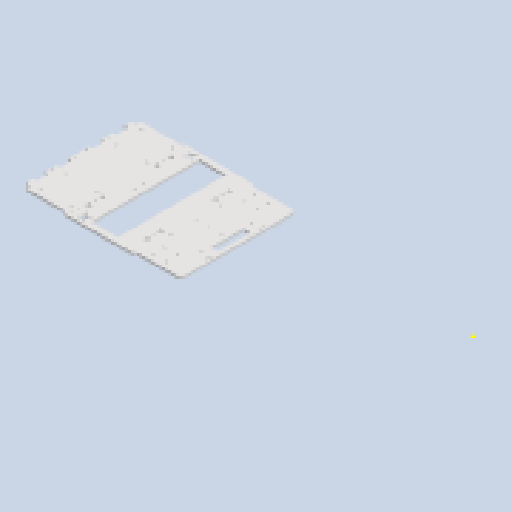
# Autodesk Inventor part: нижняя пластина
Saved by Autodesk Inventor 2024.2 (Build 282272000, 272)
## iProperties
Created: 2025-11-23
Part Number: нижняя пластина
Material: Типовые
Document SubType Name: Modeling
Designer: katya_notebook
Density: 1 g/cm^3
Appearance: По умолчанию
Author: katya_notebook
Autodesk Inventor part; units mm, degrees
(part 1 of 2)
ref_plane "YZ Plane" through (0, 0, 0) normal (1, 0, 0) x (0, 1, 0)
ref_plane "XZ Plane" through (0, 0, 0) normal (0, 1, 0) x (-1, 0, 0)
ref_plane "XY Plane" through (0, 0, 0) normal (0, 0, 1) x (1, 0, 0)
ref_plane "РабПлоскость1" through (-553.278877, -264.300199, 1.422232) normal (0, 1, 0) x (-1, 0, 0)
sketch "Эскиз1" plane through (-553.278877, -264.300199, 1.422232) normal (0, 1, 0) x (-1, 0, 0)
  line L0 (-30, 163.500004) -> (30, 163.500003)
  line L1 (-30, -31.5) -> (30, -31.5)
  line L2 (46.476267, 163.500003) -> (-223.523733, 163.500003)
  line L3 (-223.523733, 163.500003) -> (-223.523733, -31.5)
  line L4 (-223.523733, -31.5) -> (46.476267, -31.5)
  line L5 (46.476267, -31.5) -> (46.476267, 163.500003)
  point P0 (-553.278877, -1.422232)
  point P1 (-30, -30)
  point P2 (30, -30)
  point P3 (30, 162.000003)
  point P4 (-30, 162.000004)
  dimension "d1" = 270
  dimension "d6" = 0
  dimension "d7" = 0
  constraints: 8 end point, 2 coincident, 2 parallel, 1 horizontal, 1 perpendicular
  measures "d1" distance of L2.start L2.end
  measures "d6" distance from line of L4 L1.end
  measures "d7" distance from line of L2 L0.end
extrude "Выдавливание1" add sketch "Эскиз1" along normal blind 4
sketch "Эскиз2" plane through (-553.278877, -264.300199, 1.422232) normal (0, -1, 0) x (1, 0, 0)
  circle A0 centre (26, 108.500004) radius 2
  circle A1 centre (-26, 151.000003) radius 2
  circle A2 centre (26, 151.000004) radius 2
  circle A3 centre (-26, 108.500003) radius 2
  line L0 (-21.5, 122.000003) -> (-21.5, 157.000003)
  line L1 (-23.5, 122.000003) -> (-21.5, 122.000003)
  line L2 (-23.5, 157.000003) -> (-23.5, 122.000003)
  line L3 (-30, 157.000003) -> (-23.5, 157.000003)
  line L4 (-30, 157.000003) -> (-30, 103.500003)
  line L5 (-30, 103.500003) -> (30, 103.500004)
  line L6 (30, 103.500004) -> (30, 157.000004)
  line L7 (23.5, 157.000004) -> (30, 157.000004)
  line L8 (23.5, 122.000004) -> (23.5, 157.000004)
  line L9 (21.5, 122.000004) -> (23.5, 122.000004)
  line L10 (21.5, 157.000004) -> (21.5, 122.000004)
  line L11 (-21.5, 157.000003) -> (21.5, 157.000004)
  circle A4 centre (26, 23.5) radius 2
  circle A5 centre (-26, -19) radius 2
  circle A6 centre (26, -19) radius 2
  circle A7 centre (-26, 23.5) radius 2
  line L12 (-21.5, 10) -> (-21.5, -25)
  line L13 (-21.5, -25) -> (21.5, -25)
  line L14 (21.5, -25) -> (21.5, 10)
  line L15 (21.5, 10) -> (23.5, 10)
  line L16 (23.5, 10) -> (23.5, -25)
  line L17 (23.5, -25) -> (30, -25)
  line L18 (30, 28.5) -> (30, -25)
  line L19 (-30, 28.5) -> (30, 28.5)
  line L20 (-30, -25) -> (-30, 28.5)
  line L21 (-30, -25) -> (-23.5, -25)
  line L22 (-23.5, -25) -> (-23.5, 10)
  line L23 (-23.5, 10) -> (-21.5, 10)
  circle A8 centre (26, -19) radius 2
  circle A9 centre (26, 23.5) radius 2
  circle A10 centre (-26, -19) radius 2
  circle A11 centre (-26, 23.5) radius 2
  circle A12 centre (26, 108.500004) radius 2
  circle A13 centre (26, 151.000004) radius 2
  circle A14 centre (-26, 108.500003) radius 2
  circle A15 centre (-26, 151.000003) radius 2
  point P0 (553.278877, -1.422232)
  constraints: 8 centre point, 8 coincident, 8 concentric
extrude "Выдавливание2" cut sketch "Эскиз2" against normal blind 4 contours A0 | A1 | A2 | A3 | A4 | A5 | A6 | A7
sketch "Эскиз3" plane through (-553.278877, -264.300199, 1.422232) normal (0, -1, 0) x (1, 0, 0)
  spline S0 degree 3 poles (167.530647, -1.5) (167.530647, -1.675228) (167.505938, -1.863112) (167.406969, -2.216269) (167.332996, -2.381628) (167.143154, -2.701977) (167.002629, -2.869355) (166.694843, -3.139058) (166.528045, -3.241917) (165.99333, -3.490366) (165.589204, -3.533982) (164.848659, -3.417135) (164.512124, -3.257434) (164.024214, -2.845742) (163.799855, -2.568258) (163.628417, -2.126382) (163.592902, -2.011125) (163.543842, -1.762124) (163.530647, -1.627897) (163.530647, -1.372102) (163.543842, -1.237875) (163.592902, -0.988874) (163.628417, -0.873617) (163.799855, -0.431742) (164.024214, -0.154257) (164.512124, 0.257435) (164.848659, 0.417136) (165.589204, 0.533983) (165.99333, 0.490367) (166.528045, 0.241918) (166.694843, 0.139059) (167.002629, -0.130644) (167.143154, -0.298022) (167.332996, -0.618371) (167.406969, -0.78373) (167.505938, -1.136887) (167.530647, -1.324772) (167.530647, -1.5) knots -1.5971811 -1.5971811 -1.5971811 -1.5971811 -1.5446127 -1.5446127 -1.49204429 -1.49204429 -1.42257961 -1.42257961 -1.35311492 -1.35311492 -1.18239978 -1.18239978 -1.01168465 -1.01168465 -0.87532923 -0.87532923 -0.83695989 -0.83695989 -0.79859055 -0.79859055 -0.76022121 -0.76022121 -0.72185188 -0.72185188 -0.58549645 -0.58549645 -0.41478132 -0.41478132 -0.24406618 -0.24406618 -0.17460149 -0.17460149 -0.10513681 -0.10513681 -0.0525684 -0.0525684 0 0 0 0
  spline S1 degree 3 poles (190.047468, -1.5) (190.047468, -1.620288) (190.036518, -1.738724) (189.995823, -1.966144) (189.966063, -2.075131) (189.855778, -2.381563) (189.753425, -2.558671) (189.3863, -3.048352) (189.043184, -3.281704) (188.267032, -3.529213) (187.832995, -3.536652) (187.236348, -3.337829) (187.042108, -3.243447) (186.680736, -2.977295) (186.514082, -2.804962) (186.286366, -2.464282) (186.197167, -2.285548) (186.077558, -1.900195) (186.047468, -1.693486) (186.047468, -1.306513) (186.077558, -1.099804) (186.197167, -0.714451) (186.286366, -0.535718) (186.514082, -0.195037) (186.680736, -0.022705) (187.042108, 0.243448) (187.236348, 0.33783) (187.832995, 0.536653) (188.267032, 0.529214) (189.043184, 0.281704) (189.3863, 0.048353) (189.753425, -0.441328) (189.855778, -0.618437) (189.966063, -0.924868) (189.995823, -1.033855) (190.036518, -1.261275) (190.047468, -1.379712) (190.047468, -1.5) knots -1.53992103 -1.53992103 -1.53992103 -1.53992103 -1.50383465 -1.50383465 -1.46774826 -1.46774826 -1.39557548 -1.39557548 -1.21717391 -1.21717391 -1.03877234 -1.03877234 -0.96241242 -0.96241242 -0.88605249 -0.88605249 -0.8280065 -0.8280065 -0.76996052 -0.76996052 -0.71191453 -0.71191453 -0.65386854 -0.65386854 -0.57750862 -0.57750862 -0.50114869 -0.50114869 -0.32274712 -0.32274712 -0.14434556 -0.14434556 -0.07217278 -0.07217278 -0.03608639 -0.03608639 0 0 0 0
  circle A0 centre (203.047466, 23.5) radius 2
  circle A1 centre (151.047466, 23.5) radius 2
  line L0 (206.802962, 28.5) -> (146.802962, 28.5)
  line L1 (146.802962, 28.5) -> (146.802962, -25)
  line L2 (206.802962, -25) -> (206.802962, 28.5)
  line L3 (197.047468, -6.5) -> (197.047468, -25)
  line L4 (157.047468, -25) -> (157.047468, -6.5)
  line L5 (157.047468, -6.5) -> (197.047468, -6.5)
  circle A2 centre (203.047467, -19) radius 2
  circle A3 centre (151.047467, -19) radius 2
  line L6 (197.047468, -25) -> (206.802962, -25)
  line L7 (146.802962, -25) -> (157.047468, -25)
  point P0 (553.278877, -1.422232)
  point P1 (167.530647, -1.5)
  point P2 (190.047468, -1.5)
  point P3 (201.315416, -20)
  point P4 (204.779518, -20)
  point P5 (149.315416, -20)
  point P6 (152.779518, -20)
extrude "Выдавливание3" cut sketch "Эскиз3" against normal blind 10 contours S0 | S1 | A0 | A1
sketch "Эскиз4" plane through (-553.278877, -264.300199, 1.422232) normal (0, -1, 0) x (1, 0, 0)
  circle A0 centre (151.047466, 108.500004) radius 2
  circle A1 centre (203.047466, 108.500003) radius 2
  spline S0 degree 3 poles (190.047468, 133.500003) (190.047468, 133.620291) (190.036518, 133.738728) (189.995823, 133.966148) (189.966063, 134.075135) (189.855778, 134.381566) (189.753425, 134.558675) (189.3863, 135.048356) (189.043184, 135.281707) (188.267032, 135.529217) (187.832995, 135.536656) (187.236348, 135.337833) (187.042108, 135.243451) (186.680736, 134.977298) (186.514082, 134.804966) (186.286366, 134.464285) (186.197167, 134.285552) (186.077558, 133.900199) (186.047468, 133.69349) (186.047468, 133.306517) (186.077558, 133.099808) (186.197167, 132.714455) (186.286366, 132.535721) (186.514082, 132.195041) (186.680736, 132.022708) (187.042108, 131.756556) (187.236348, 131.662174) (187.832995, 131.46335) (188.267032, 131.47079) (189.043184, 131.718299) (189.3863, 131.95165) (189.753425, 132.441332) (189.855778, 132.61844) (189.966063, 132.924872) (189.995823, 133.033859) (190.036518, 133.261279) (190.047468, 133.379715) (190.047468, 133.500003) knots 0 0 0 0 0.03608639 0.03608639 0.07217278 0.07217278 0.14434556 0.14434556 0.32274712 0.32274712 0.50114869 0.50114869 0.57750862 0.57750862 0.65386854 0.65386854 0.71191453 0.71191453 0.76996052 0.76996052 0.8280065 0.8280065 0.88605249 0.88605249 0.96241242 0.96241242 1.03877234 1.03877234 1.21717391 1.21717391 1.39557548 1.39557548 1.46774826 1.46774826 1.50383465 1.50383465 1.53992103 1.53992103 1.53992103 1.53992103
  spline S1 degree 3 poles (167.530647, 133.500003) (167.530647, 133.675231) (167.505938, 133.863116) (167.406969, 134.216273) (167.332996, 134.381632) (167.143154, 134.701981) (167.002629, 134.869359) (166.694843, 135.139062) (166.528045, 135.241921) (165.99333, 135.49037) (165.589204, 135.533986) (164.848659, 135.417139) (164.512124, 135.257438) (164.024214, 134.845746) (163.799855, 134.568261) (163.628417, 134.126386) (163.592902, 134.011129) (163.543842, 133.762128) (163.530647, 133.627901) (163.530647, 133.372105) (163.543842, 133.237879) (163.592902, 132.988878) (163.628417, 132.873621) (163.799855, 132.431745) (164.024214, 132.154261) (164.512124, 131.742569) (164.848659, 131.582868) (165.589204, 131.466021) (165.99333, 131.509637) (166.528045, 131.758086) (166.694843, 131.860945) (167.002629, 132.130648) (167.143154, 132.298026) (167.332996, 132.618375) (167.406969, 132.783734) (167.505938, 133.136891) (167.530647, 133.324775) (167.530647, 133.500003) knots 0 0 0 0 0.0525684 0.0525684 0.10513681 0.10513681 0.17460149 0.17460149 0.24406618 0.24406618 0.41478132 0.41478132 0.58549645 0.58549645 0.72185188 0.72185188 0.76022121 0.76022121 0.79859055 0.79859055 0.83695989 0.83695989 0.87532923 0.87532923 1.01168465 1.01168465 1.18239978 1.18239978 1.35311492 1.35311492 1.42257961 1.42257961 1.49204429 1.49204429 1.5446127 1.5446127 1.5971811 1.5971811 1.5971811 1.5971811
  circle A2 centre (151.047467, 151.000004) radius 2
  circle A3 centre (203.047467, 151.000003) radius 2
  point P0 (553.278877, -1.422232)
  point P1 (190.047468, 133.500003)
  point P2 (167.530647, 133.500003)
  point P3 (149.315416, 152.000003)
  point P4 (152.779518, 152.000003)
  point P5 (201.315416, 152.000003)
  point P6 (204.779518, 152.000003)
extrude "Выдавливание4" cut sketch "Эскиз4" against normal blind 10 contours A0 | A1 | S0 | S1
sketch "Эскиз6" plane through (-553.278877, -264.300199, 1.422232) normal (0, -1, 0) x (1, 0, 0)
  circle A0 centre (53.523733, 156.000002) radius 5
  circle A1 centre (53.523733, 156.000002) radius 2.5
  circle A2 centre (53.523733, 156.000002) radius 5
  circle A3 centre (53.523733, -23.999998) radius 5
  circle A4 centre (53.523733, -23.999998) radius 5
  point P0 (553.278877, -1.422232)
  constraints: 2 centre point, 2 coincident, 2 concentric
extrude "Выдавливание6" cut sketch "Эскиз6" against normal blind 10 contours A0 | A1 | A3
sketch "Эскиз7" plane through (-553.278877, -264.300199, 1.422232) normal (0, -1, 0) x (1, 0, 0)
  line L0 (30, 103.500004) -> (30, 157.000004)
  line L1 (-46.476267, 163.500003) -> (223.523733, 163.500003)
  line L2 (30.270127, 167.770131) -> (146.697322, 167.770131)
  line L3 (146.802962, 163.500003) -> (146.802962, 157.000003)
  line L4 (146.802962, 167.770131) -> (146.697322, 167.770131)
  line L5 (146.802962, 163.500003) -> (30, 163.500003)
  line L6 (30.000003, 28.5) -> (30.000003, -25)
  line L7 (30.000003, -25) -> (30.000003, -31.5)
  line L8 (146.802962, -31.5) -> (146.802962, -25)
  line L9 (146.802962, -35.5) -> (30.000003, -35.5)
  line L10 (30.000003, -31.5) -> (146.802962, -31.5)
  line L11 (30, 163.500003) -> (26, 163.500003)
  arc A0 (26, 163.500003) -> (30.270127, 167.770131) centre (22.8966, 170.873531) ccw
  line L12 (146.802962, 163.500003) -> (150.802962, 163.500003)
  arc A1 (146.802962, 167.770131) -> (150.802962, 163.500003) centre (154.237087, 170.72543) ccw
  line L13 (30.000003, -31.5) -> (26.000003, -31.5)
  line L14 (223.523733, -31.5) -> (-46.476267, -31.5)
  arc A2 (30.000003, -35.5) -> (26.000003, -31.5) centre (22.7085, -38.791502) ccw
  line L15 (146.802962, -31.5) -> (150.802962, -31.5)
  arc A3 (150.802962, -31.5) -> (146.802962, -35.5) centre (154.094465, -38.791502) ccw
  point P0 (553.278877, -1.422232)
  dimension "d23" = 8
  dimension "d24" = 8
  dimension "d26" = 8
  dimension "d28" = 8
  constraints: 18 end point, 8 point on circle, 5 point on line, 4 centre point, 2 collinear, 1 parallel
  measures "d23" radius of A0
  measures "d24" radius of A1
  measures "d26" radius of A2
  measures "d28" radius of A3
extrude "Выдавливание7" add sketch "Эскиз7" against normal blind 4
sketch "Эскиз8" plane through (-553.278877, -264.300199, 1.422232) normal (0, -1, 0) x (1, 0, 0)
  circle A0 centre (57.777238, 162.775524) radius 1.5
  circle A1 centre (60.299256, 151.746498) radius 1.5
  circle A2 centre (49.270229, 149.22448) radius 1.5
  circle A3 centre (46.748211, 160.253506) radius 1.5
  circle A4 centre (57.777238, 162.775524) radius 1.5
  circle A5 centre (60.299256, 151.746498) radius 1.5
  circle A6 centre (49.270229, 149.22448) radius 1.5
  circle A7 centre (46.748211, 160.253506) radius 1.5
  circle A8 centre (60.299256, -19.746494) radius 1.5
  circle A9 centre (57.777238, -30.775521) radius 1.5
  circle A10 centre (46.748211, -28.253503) radius 1.5
  circle A11 centre (49.270229, -17.224476) radius 1.5
  circle A12 centre (49.270229, -17.224476) radius 1.5
  circle A13 centre (60.299256, -19.746494) radius 1.5
  circle A14 centre (57.777238, -30.775521) radius 1.5
  circle A15 centre (46.748211, -28.253503) radius 1.5
  point P0 (553.278877, -1.422232)
  constraints: 8 centre point, 8 coincident, 8 concentric
extrude "Выдавливание8" cut sketch "Эскиз8" against normal blind 4
sketch "Эскиз9" plane through (-553.278877, -264.300199, 1.422232) normal (0, -1, 0) x (1, 0, 0)
  line L0 (223.523733, 163.500003) -> (223.523733, -31.5)
  line L1 (-46.476267, -31.5) -> (-46.476267, 163.500003)
  line L2 (223.523733, 163.500003) -> (-46.476267, 163.500003)
  line L3 (-46.476267, 163.500003) -> (-46.476267, -31.5)
  line L4 (-46.476267, -31.5) -> (223.523733, -31.5)
  line L5 (223.523733, -31.5) -> (223.523733, 163.500003)
  line L6 (223.523733, 66.000002) -> (-46.476267, 66.000002)
  line L7 (88.523733, 163.500003) -> (88.523733, -31.5)
  line L8 (66.023733, -25.499998) -> (111.023733, -25.499998)
  line L9 (111.023733, -25.499998) -> (111.023733, 157.500002)
  line L10 (111.023733, 157.500002) -> (66.023733, 157.500002)
  line L11 (66.023733, 157.500002) -> (66.023733, -25.499998)
  line L12 (66.023733, -25.499998) -> (111.023733, 157.500002) construction
  line L13 (111.023733, -25.499998) -> (66.023733, 157.500002) construction
  point P0 (553.278877, -1.422232)
  point P1 (88.523733, 66.000002)
  dimension "d33" = 183
  dimension "d34" = 45
  constraints: 24 end point, 7 midpoint, 4 parallel, 2 horizontal, 2 perpendicular
  measures "d33" distance of L8.end L9.end
  measures "d34" distance of L9.end L10.end
extrude "Выдавливание9" cut sketch "Эскиз9" against normal blind 4 contours L9 L8 L7 L6 | L6 L7 L10 L9 | L7 L6 L11 L10 | L7 L8 L11 L6
sketch "Эскиз10" plane through (-553.278877, -264.300199, 1.422232) normal (0, -1, 0) x (1, 0, 0)
  line L0 (36.973733, 147.850002) -> (34.973733, 147.850002)
  line L1 (36.973733, 147.850002) -> (36.973733, 152.650002)
  line L2 (35.973733, 147.850002) -> (35.973733, 152.650002)
  line L3 (36.973733, 159.350002) -> (34.973733, 159.350002)
  line L4 (36.973733, 150.250002) -> (34.973733, 150.250002)
  line L5 (36.973733, 159.350002) -> (36.973733, 164.150002)
  line L6 (36.973733, 161.750002) -> (33.994288, 161.750002)
  line L7 (33.994288, 161.750002) -> (35.973733, 159.350002)
  line L8 (35.973733, 164.150002) -> (35.973733, 159.350002)
  circle A0 centre (35.973733, 161.750002) radius 1
  circle A1 centre (35.973733, 150.250002) radius 1
  point P0 (553.278877, -1.422232)
  point P1 (34.973733, 147.000002)
  point P2 (30, 163.500005)
  point P3 (34.973733, 161.750002)
  point P4 (35.973733, 162.750002)
  point P5 (35.973733, 161.750002)
  constraints: 18 end point, 4 midpoint, 4 perpendicular, 2 horizontal, 1 horizontal alignment, 6 other
extrude "Выдавливание10" cut sketch "Эскиз10" against normal blind 10 contours A1 L2 L4 | L4 L2 A1 | A1 L4 L2 | L4 A1 L2 | A0 L8 L6 | L6 L8 A0 | A0 L6 L8 | L6 A0 L8
sketch "Эскиз11" plane through (-553.278877, -264.300199, 1.422232) normal (0, -1, 0) x (1, 0, 0)
  arc A0 (34.973733, -29.749998) -> (36.973733, -29.749998) centre (35.973733, -29.749998) ccw
  arc A1 (36.973733, -29.749998) -> (34.973733, -29.749998) centre (35.973733, -29.749998) ccw
  arc A2 (34.973733, -18.249998) -> (36.973733, -18.249998) centre (35.973733, -18.249998) ccw
  arc A3 (36.973733, -18.249998) -> (34.973733, -18.249998) centre (35.973733, -18.249998) ccw
  point P0 (553.278877, -1.422232)
extrude "Выдавливание11" cut sketch "Эскиз11" against normal blind 10
sketch "Эскиз12" plane through (-553.278877, -264.300199, 1.422232) normal (0, -1, 0) x (1, 0, 0)
  circle A0 centre (55.548733, 57.85394) radius 2
  circle A1 centre (55.548733, 73.85394) radius 2
  point P0 (553.278877, -1.422232)
extrude "Выдавливание12" cut sketch "Эскиз12" against normal blind 10
sketch "Эскиз13" plane through (-553.278877, -264.300199, 1.422232) normal (0, -1, 0) x (1, 0, 0)
  point P0 (553.278877, -1.422232)
sketch "Эскиз14" plane through (-553.278877, -264.300199, 1.422232) normal (0, -1, 0) x (1, 0, 0)
  circle A0 centre (217.523733, 18.5) radius 2
  circle A1 centre (217.523733, 113.500003) radius 2
  line L0 (150.802962, 163.500003) -> (223.523733, 163.500003)
  line L1 (223.523733, -31.5) -> (150.802962, -31.5)
  line L2 (223.523733, 163.500003) -> (223.523733, -31.5)
  circle A2 centre (217.523733, 24.5) radius 2
  circle A3 centre (217.523733, 107.500003) radius 2
  point P0 (553.278877, -1.422232)
  dimension "d43" = 4
  dimension "d44" = 4
  dimension "d45" = 50
  dimension "d46" = 50
  dimension "d47" = 6
  dimension "d48" = 6
  dimension "d51" = 4
  dimension "d52" = 6
  dimension "d53" = 6
  dimension "d54" = 4
  dimension "d55" = 6
  dimension "d56" = 6
  constraints: 4 centre point
  measures "d43" diameter of A1
  measures "d44" diameter of A0
  measures "d45" distance from line of L0 A1.centre
  measures "d46" distance from line of L1 A0.centre
  measures "d47" distance from line of L2 A0.centre
  measures "d48" distance from line of L2 A1.centre
  measures "d51" diameter of A3
  measures "d52" distance of A1.centre A3.centre
  measures "d53" distance from line of L2 A3.centre
  measures "d54" diameter of A2
  measures "d55" distance from line of L2 A2.centre
  measures "d56" distance of A0.centre A2.centre
extrude "Выдавливание13" cut sketch "Эскиз14" against normal blind 10
sketch "Эскиз15" plane through (-553.278877, -264.300199, 1.422232) normal (0, -1, 0) x (1, 0, 0)
  line L0 (216.523733, 93.576493) -> (204.523733, 93.576493)
  line L1 (204.523733, 93.576493) -> (204.523733, 38.576493)
  line L2 (204.523733, 38.576493) -> (216.523733, 38.576493)
  line L3 (216.523733, 38.576493) -> (216.523733, 93.576493)
  line L4 (216.523733, 93.576493) -> (204.523733, 38.576493) construction
  line L5 (204.523733, 93.576493) -> (216.523733, 38.576493) construction
  line L6 (223.523733, 163.500003) -> (223.523733, -31.5)
  point P0 (553.278877, -1.422232)
  point P1 (210.523733, 66.076493)
  dimension "d57" = 13
  dimension "d58" = 12
  dimension "d59" = 55
  constraints: 12 end point, 2 midpoint, 2 parallel, 1 horizontal, 1 perpendicular
  measures "d57" distance from line of point (210.524, 66.076) L6
  measures "d58" distance of L0.start L0.end
  measures "d59" distance of L0.end L1.end
extrude "Выдавливание14" cut sketch "Эскиз15" against normal blind 10
sketch "Эскиз16" plane through (-553.278877, -264.300199, 1.422232) normal (0, -1, 0) x (1, 0, 0)
  spline S0 degree 3 poles (195.773733, 65.9) (195.773733, 66.088725) (195.735944, 66.289784) (195.582756, 66.659245) (195.467375, 66.827679) (195.201416, 67.093638) (195.03298, 67.209022) (194.663513, 67.362213) (194.462453, 67.4) (194.085014, 67.4) (193.883953, 67.362213) (193.514486, 67.209022) (193.346051, 67.093638) (193.080092, 66.827679) (192.964711, 66.659245) (192.811522, 66.289784) (192.773733, 66.088725) (192.773733, 65.711276) (192.811522, 65.510217) (192.964711, 65.140756) (193.080092, 64.972321) (193.346051, 64.706363) (193.514486, 64.590979) (193.883953, 64.437788) (194.085014, 64.4) (194.462453, 64.4) (194.663513, 64.437788) (195.03298, 64.590979) (195.201416, 64.706363) (195.467375, 64.972321) (195.582756, 65.140756) (195.735944, 65.510217) (195.773733, 65.711276) (195.773733, 65.9) knots -0.905867 -0.905867 -0.905867 -0.905867 -0.84924956 -0.84924956 -0.79263212 -0.79263212 -0.73601619 -0.73601619 -0.67940025 -0.67940025 -0.62278432 -0.62278432 -0.56616839 -0.56616839 -0.50955095 -0.50955095 -0.4529335 -0.4529335 -0.39631606 -0.39631606 -0.33969861 -0.33969861 -0.28308268 -0.28308268 -0.22646675 -0.22646675 -0.16985082 -0.16985082 -0.11323489 -0.11323489 -0.05661744 -0.05661744 0 0 0 0
  spline S1 degree 3 poles (172.273733, 66.1) (172.273733, 65.911276) (172.311522, 65.710217) (172.464711, 65.340756) (172.580092, 65.172321) (172.846051, 64.906363) (173.014486, 64.790979) (173.383953, 64.637788) (173.585014, 64.6) (173.962453, 64.6) (174.163513, 64.637788) (174.53298, 64.790979) (174.701416, 64.906363) (174.967375, 65.172321) (175.082756, 65.340756) (175.235944, 65.710217) (175.273733, 65.911276) (175.273733, 66.288725) (175.235944, 66.489784) (175.082756, 66.859245) (174.967375, 67.027679) (174.701416, 67.293638) (174.53298, 67.409022) (174.163513, 67.562213) (173.962453, 67.6) (173.585014, 67.6) (173.383953, 67.562213) (173.014486, 67.409022) (172.846051, 67.293638) (172.580092, 67.027679) (172.464711, 66.859245) (172.311522, 66.489784) (172.273733, 66.288725) (172.273733, 66.1) knots -0.905867 -0.905867 -0.905867 -0.905867 -0.84924956 -0.84924956 -0.79263212 -0.79263212 -0.73601619 -0.73601619 -0.67940025 -0.67940025 -0.62278432 -0.62278432 -0.56616839 -0.56616839 -0.50955095 -0.50955095 -0.4529335 -0.4529335 -0.39631606 -0.39631606 -0.33969861 -0.33969861 -0.28308268 -0.28308268 -0.22646675 -0.22646675 -0.16985082 -0.16985082 -0.11323489 -0.11323489 -0.05661744 -0.05661744 0 0 0 0
  spline S2 degree 3 poles (154.773733, 65.9) (154.773733, 66.088725) (154.735944, 66.289784) (154.582756, 66.659245) (154.467375, 66.827679) (154.201416, 67.093638) (154.03298, 67.209022) (153.663513, 67.362213) (153.462453, 67.4) (153.085014, 67.4) (152.883953, 67.362213) (152.514486, 67.209022) (152.346051, 67.093638) (152.080092, 66.827679) (151.964711, 66.659245) (151.811522, 66.289784) (151.773733, 66.088725) (151.773733, 65.711276) (151.811522, 65.510217) (151.964711, 65.140756) (152.080092, 64.972321) (152.346051, 64.706363) (152.514486, 64.590979) (152.883953, 64.437788) (153.085014, 64.4) (153.462453, 64.4) (153.663513, 64.437788) (154.03298, 64.590979) (154.201416, 64.706363) (154.467375, 64.972321) (154.582756, 65.140756) (154.735944, 65.510217) (154.773733, 65.711276) (154.773733, 65.9) knots -0.905867 -0.905867 -0.905867 -0.905867 -0.84924956 -0.84924956 -0.79263212 -0.79263212 -0.73601619 -0.73601619 -0.67940025 -0.67940025 -0.62278432 -0.62278432 -0.56616839 -0.56616839 -0.50955095 -0.50955095 -0.4529335 -0.4529335 -0.39631606 -0.39631606 -0.33969861 -0.33969861 -0.28308268 -0.28308268 -0.22646675 -0.22646675 -0.16985082 -0.16985082 -0.11323489 -0.11323489 -0.05661744 -0.05661744 0 0 0 0
  point P0 (553.278877, -1.422232)
  point P1 (195.773733, 65.9)
  point P2 (172.273733, 66.1)
  point P3 (154.773733, 65.9)
extrude "Выдавливание15" cut sketch "Эскиз16" against normal blind 10
sketch "Эскиз17" plane through (-553.278877, -260.300199, 1.422232) normal (0, 1, 0) x (1, 0, 0)
  line L0 (-46.476267, -143.500003) -> (-46.476267, -123.500003)
  line L1 (-46.476267, -143.500003) -> (-40.476267, -143.500003)
  line L2 (-40.476267, -123.500003) -> (-40.476267, -143.500003)
  line L3 (-46.476267, -123.500003) -> (-40.476267, -123.500003)
  line L4 (-46.476267, -103.500003) -> (-46.476267, -83.500003)
  line L5 (-46.476267, -103.500003) -> (-40.476267, -103.500003)
  line L6 (-40.476267, -83.500003) -> (-40.476267, -103.500003)
  line L7 (-46.476267, -83.500003) -> (-40.476267, -83.500003)
  line L8 (-46.476267, -48.5) -> (-46.476267, -28.5)
  line L9 (-46.476267, -48.5) -> (-40.476267, -48.5)
  line L10 (-40.476267, -28.5) -> (-40.476267, -48.5)
  line L11 (-46.476267, -28.5) -> (-40.476267, -28.5)
  line L12 (-46.476267, -8.5) -> (-46.476267, 11.5)
  line L13 (-46.476267, -8.5) -> (-40.476267, -8.5)
  line L14 (-40.476267, 11.5) -> (-40.476267, -8.5)
  line L15 (-46.476267, 11.5) -> (-40.476267, 11.5)
  circle A0 centre (-43.476267, -113.500003) radius 1.75
  circle A1 centre (-43.476267, -76.375003) radius 1.75
  circle A2 centre (-43.476267, -55.625003) radius 1.75
  circle A3 centre (-43.476267, -18.5) radius 1.75
  point P0 (553.278877, 1.422232)
extrude "Выдавливание16" cut sketch "Эскиз17" against normal blind 10
fillet "Сопряжение1" radius 8 4 edges at (-329.7551, -262.3002, -30.0778) (-329.7551, -262.3002, 164.9222) (-599.7551, -262.3002, -30.0778) (-599.7551, -262.3002, 164.9222)
sketch "Эскиз18" plane through (-599.755143, -264.300199, 104.922235) normal (-1, 0, 0) x (0, 0, 1)
  line L0 (-95.000003, 0) -> (-95.000003, 4)
  line L1 (-95.000003, 4) -> (-95.000003, 5)
  line L2 (-95.000003, 5) -> (-115.000003, 5)
  line L3 (-115.000003, 5) -> (-115.000003, 4)
  line L4 (-135.000003, 4) -> (-127.000003, 4)
  line L5 (-135.000003, 4) -> (-135.000003, -55.704973)
  line L6 (-115.000003, -55.704973) -> (-135.000003, -55.704973)
  line L7 (-115.000003, -55.704973) -> (-115.000003, -60.704973)
  line L8 (-115.000003, -60.704973) -> (-95.000003, -60.704973)
  line L9 (-95.000003, -60.704973) -> (-95.000003, -55.704973)
  line L10 (-86.750003, -55.704973) -> (-95.000003, -55.704973)
  line L11 (-86.750003, -55.704973) -> (-86.750003, -54.204972)
  line L12 (-86.750003, -54.204972) -> (-88.250003, -54.204972)
  line L13 (-88.250003, -54.204972) -> (-88.250003, -51.204972)
  line L14 (-88.250003, -51.204972) -> (-86.750003, -51.204972)
  line L15 (-86.750003, -51.204972) -> (-86.750003, -43.704972)
  line L16 (-86.750003, -43.704972) -> (-83.250003, -43.704972)
  line L17 (-83.250003, -43.704972) -> (-83.250003, -51.204972)
  line L18 (-83.250003, -51.204972) -> (-81.750003, -51.204972)
  line L19 (-81.750003, -51.204972) -> (-81.750003, -54.204972)
  line L20 (-81.750003, -54.204972) -> (-83.250003, -54.204972)
  line L21 (-83.250003, -54.204972) -> (-83.250003, -55.704973)
  line L22 (-75.000003, -55.704973) -> (-83.250003, -55.704973)
  line L23 (-75.000003, -55.704973) -> (-75.000003, -60.704973)
  line L24 (-75.000003, -60.704973) -> (-55.000003, -60.704972)
  line L25 (-55.000003, -60.704972) -> (-55.000003, -55.704972)
  line L26 (-49.624972, -55.704972) -> (-55.000003, -55.704972)
  line L27 (-49.624972, -55.704972) -> (-49.624972, -54.204972)
  line L28 (-49.624972, -54.204972) -> (-51.124972, -54.204972)
  line L29 (-51.124972, -54.204972) -> (-51.124972, -51.204972)
  line L30 (-51.124972, -51.204972) -> (-49.624972, -51.204972)
  line L31 (-49.624972, -51.204972) -> (-49.624972, -49.704972)
  line L32 (-49.624972, -49.704972) -> (-49.625, -49.704972)
  line L33 (-49.625, -49.704972) -> (-49.625, -43.704972)
  line L34 (-49.625, -43.704972) -> (-46.124972, -43.704972)
  line L35 (-46.124972, -43.704972) -> (-46.124972, -51.204972)
  line L36 (-46.124972, -51.204972) -> (-44.624972, -51.204972)
  line L37 (-44.624972, -51.204972) -> (-44.624972, -54.204972)
  line L38 (-44.624972, -54.204972) -> (-46.124972, -54.204972)
  line L39 (-46.124972, -54.204972) -> (-46.124972, -55.704972)
  line L40 (-28.875, -55.704972) -> (-46.124972, -55.704972)
  line L41 (-28.875, -55.704972) -> (-28.875, -54.204972)
  line L42 (-28.875, -54.204972) -> (-30.375, -54.204972)
  line L43 (-30.375, -54.204972) -> (-30.375, -51.204972)
  line L44 (-30.375, -51.204972) -> (-28.875, -51.204972)
  line L45 (-28.875, -51.204972) -> (-28.875, -43.704972)
  line L46 (-28.875, -43.704972) -> (-25.375, -43.704972)
  line L47 (-25.375, -43.704972) -> (-25.375, -51.204972)
  line L48 (-25.375, -51.204972) -> (-23.875, -51.204972)
  line L49 (-23.875, -51.204972) -> (-23.875, -54.204972)
  line L50 (-23.875, -54.204972) -> (-25.375, -54.204972)
  line L51 (-25.375, -54.204972) -> (-25.375, -55.704972)
  line L52 (-20, -55.704972) -> (-25.375, -55.704972)
  line L53 (-20, -55.704972) -> (-20, -60.704972)
  line L54 (-20, -60.704972) -> (0, -60.704972)
  line L55 (0, -60.704972) -> (0, -55.704972)
  line L56 (8.25, -55.704972) -> (0, -55.704972)
  line L57 (8.25, -55.704972) -> (8.25, -54.204972)
  line L58 (8.25, -54.204972) -> (6.75, -54.204972)
  line L59 (6.75, -54.204972) -> (6.75, -51.204972)
  line L60 (6.75, -51.204972) -> (8.25, -51.204972)
  line L61 (8.25, -51.204972) -> (8.25, -43.704972)
  line L62 (8.25, -43.704972) -> (11.75, -43.704972)
  line L63 (11.75, -43.704972) -> (11.75, -51.204972)
  line L64 (11.75, -51.204972) -> (13.25, -51.204972)
  line L65 (13.25, -51.204972) -> (13.25, -54.204972)
  line L66 (13.25, -54.204972) -> (11.75, -54.204972)
  line L67 (11.75, -54.204972) -> (11.75, -55.704972)
  line L68 (20, -55.704972) -> (11.75, -55.704972)
  line L69 (20, -55.704972) -> (20, -60.704972)
  line L70 (20, -60.704972) -> (40, -60.704972)
  line L71 (40, -60.704972) -> (40, -55.704972)
  line L72 (60, -55.704972) -> (40, -55.704972)
  line L73 (60, 4) -> (60, -55.704972)
  line L74 (52, 4) -> (60, 4)
  line L75 (40, 4) -> (40, 5)
  line L76 (40, 5) -> (20, 5)
  line L77 (20, 5) -> (20, 4)
  line L78 (20, 4) -> (20, 0)
  line L79 (20, 0) -> (13.25, 0)
  line L80 (13.25, 0) -> (13.25, -0.5)
  line L81 (13.25, -0.5) -> (11.75, -0.5)
  line L82 (11.75, -0.5) -> (11.75, -8)
  line L83 (11.75, -8) -> (8.25, -8)
  line L84 (8.25, -8) -> (8.25, -0.5)
  line L85 (8.25, -0.5) -> (6.75, -0.5)
  line L86 (6.75, -0.5) -> (6.75, 0)
  line L87 (6.75, 0) -> (0, 0)
  line L88 (0, 0) -> (0, 4)
  line L89 (0, 4) -> (0, 5)
  line L90 (0, 5) -> (-20, 5)
  line L91 (-20, 5) -> (-20, 4)
  line L92 (-20, 4) -> (-20, 0)
  line L93 (-20, 0) -> (-23.875, 0)
  line L94 (-23.875, 0) -> (-23.875, -0.5)
  line L95 (-23.875, -0.5) -> (-25.375, -0.5)
  line L96 (-25.375, -0.5) -> (-25.375, -8)
  line L97 (-25.375, -8) -> (-28.875, -8)
  line L98 (-28.875, -8) -> (-28.875, -0.5)
  line L99 (-28.875, -0.5) -> (-30.375, -0.5)
  line L100 (-30.375, -0.5) -> (-30.375, 0)
  line L101 (-30.375, 0) -> (-44.624972, 0)
  line L102 (-44.624972, 0) -> (-44.624972, -0.5)
  line L103 (-44.624972, -0.5) -> (-46.124972, -0.5)
  line L104 (-46.124972, -0.5) -> (-46.124972, -8)
  line L105 (-46.124972, -8) -> (-49.625, -8)
  line L106 (-49.625, -8) -> (-49.625, -2)
  line L107 (-49.625, -2) -> (-49.624972, -2)
  line L108 (-49.624972, -2) -> (-49.624972, -0.5)
  line L109 (-49.624972, -0.5) -> (-51.124972, -0.5)
  line L110 (-51.124972, -0.5) -> (-51.124972, 0)
  line L111 (-51.124972, 0) -> (-55.000003, 0)
  line L112 (-55.000003, 0) -> (-55.000003, 4)
  line L113 (-55.000003, 4) -> (-55.000003, 5)
  line L114 (-55.000003, 5) -> (-75.000003, 5)
  line L115 (-75.000003, 5) -> (-75.000003, 4)
  line L116 (-75.000003, 4) -> (-75.000003, 0)
  line L117 (-75.000003, 0) -> (-81.750003, 0)
  line L118 (-81.750003, 0) -> (-81.750003, -0.5)
  line L119 (-81.750003, -0.5) -> (-83.250003, -0.5)
  line L120 (-83.250003, -0.5) -> (-83.250003, -8)
  line L121 (-83.250003, -8) -> (-86.750003, -8)
  line L122 (-86.750003, -8) -> (-86.750003, -0.5)
  line L123 (-86.750003, -0.5) -> (-88.250003, -0.5)
  line L124 (-88.250003, -0.5) -> (-88.250003, 0)
  line L125 (-88.250003, 0) -> (-95.000003, 0)
  line L126 (52, 0) -> (-127.000003, 0)
  line L127 (52, 0) -> (52, 4)
  line L128 (52, 4) -> (60, 4)
  line L129 (60, 0) -> (60, 4)
  line L130 (60, 0) -> (52, 0)
  line L131 (-127.000003, 0) -> (-127.000003, 4)
  line L132 (-135.000003, 0) -> (-135.000003, 4)
  line L133 (-127.000003, 4) -> (-135.000003, 4)
  line L134 (-135.000003, 0) -> (-127.000003, 0)
  line L135 (-127.000003, 0) -> (-127.000003, 4)
  line L136 (52, 4) -> (52, 0)
  line L137 (52, 0) -> (40, 0)
  line L138 (40, 0) -> (40, 4)
  line L139 (-115.000003, 4) -> (-115.000003, 0)
  line L140 (-115.000003, 0) -> (-127.000003, 0)
  line L141 (-86.23393, -29.706046) -> (-86.23393, -22.248836)
  spline S0 degree 2 poles (-86.23393, -22.248836) (-86.23393, -21.656701) (-85.641794, -21.656701) knots 0 0 0 1 1 1
  spline S1 degree 2 poles (-85.641794, -21.656701) (-85.049659, -21.656701) (-85.049659, -22.248836) knots 0 0 0 1 1 1
  line L142 (-85.049659, -22.248836) -> (-85.049659, -29.11391)
  line L143 (-85.049659, -29.11391) -> (-83.624832, -29.11391)
  line L144 (-83.624832, -29.11391) -> (-82.051972, -22.054542)
  spline S2 degree 2 poles (-82.051972, -22.054542) (-81.95945, -21.656701) (-81.496844, -21.656701) knots 0 0 0 1 1 1
  spline S3 degree 2 poles (-81.496844, -21.656701) (-80.904709, -21.656701) (-80.904709, -22.230332) knots 0 0 0 1 1 1
  spline S4 degree 2 poles (-80.904709, -22.230332) (-80.904709, -22.304349) (-80.913961, -22.359862) knots 0 0 0 1 1 1
  line L145 (-80.913961, -22.359862) -> (-82.588595, -29.90034)
  spline S5 degree 2 poles (-82.588595, -29.90034) (-82.681116, -30.288929) (-83.152974, -30.288929) knots 0 0 0 1 1 1
  line L146 (-83.152974, -30.288929) -> (-85.641794, -30.288929)
  spline S6 degree 2 poles (-85.641794, -30.288929) (-86.23393, -30.288929) (-86.23393, -29.706046) knots 0 0 0 1 1 1
  line L147 (-79.442874, -28.466261) -> (-79.442874, -23.488621)
  spline S7 degree 2 poles (-79.442874, -23.488621) (-79.442874, -22.729947) (-78.369628, -21.656701) (-77.610954, -21.656701) knots 0 0 0 1 2 2 2
  line L148 (-77.610954, -21.656701) -> (-75.954824, -21.656701)
  spline S8 degree 2 poles (-75.954824, -21.656701) (-75.186898, -21.656701) (-74.122904, -22.729947) (-74.122904, -23.488621) knots 0 0 0 1 2 2 2
  line L149 (-74.122904, -23.488621) -> (-74.122904, -28.466261)
  spline S9 degree 2 poles (-74.122904, -28.466261) (-74.122904, -29.215683) (-75.19615, -30.288929) (-75.954824, -30.288929) knots 0 0 0 1 2 2 2
  line L150 (-75.954824, -30.288929) -> (-77.610954, -30.288929)
  spline S10 degree 2 poles (-77.610954, -30.288929) (-78.360376, -30.288929) (-79.442874, -29.206431) (-79.442874, -28.466261) knots 0 0 0 1 2 2 2
  spline S11 degree 2 poles (-44.950968, -30.270425) (-45.200775, -30.270425) (-45.561608, -29.909592) (-45.561608, -29.678289) knots 0 0 0 1 2 2 2
  spline S12 degree 2 poles (-45.561608, -29.678289) (-45.561608, -29.46549) (-45.404322, -29.2897) knots 0 0 0 1 1 1
  spline S13 degree 2 poles (-45.404322, -29.2897) (-44.109025, -27.864874) (-42.878493, -26.560325) knots 0 0 0 1 1 1
  line L151 (-42.878493, -26.560325) -> (-45.450582, -22.554156)
  spline S14 degree 2 poles (-45.450582, -22.554156) (-45.543104, -22.406122) (-45.543104, -22.248836) knots 0 0 0 1 1 1
  spline S15 degree 2 poles (-45.543104, -22.248836) (-45.543104, -21.999029) (-45.173019, -21.656701) (-44.941716, -21.656701) knots 0 0 0 1 2 2 2
  spline S16 degree 2 poles (-44.941716, -21.656701) (-44.636396, -21.656701) (-44.432849, -22.063794) knots 0 0 0 1 1 1
  line L152 (-44.432849, -22.063794) -> (-42.101315, -25.764642)
  spline S17 degree 2 poles (-42.101315, -25.764642) (-42.027298, -25.561096) (-41.398154, -24.867187) knots 0 0 0 1 1 1
  line L153 (-41.398154, -24.867187) -> (-41.398154, -22.248836)
  spline S18 degree 2 poles (-41.398154, -22.248836) (-41.398154, -21.656701) (-40.806018, -21.656701) knots 0 0 0 1 1 1
  spline S19 degree 2 poles (-40.806018, -21.656701) (-40.213882, -21.656701) (-40.213882, -22.248836) knots 0 0 0 1 1 1
  line L154 (-40.213882, -22.248836) -> (-40.213882, -29.706046)
  spline S20 degree 2 poles (-40.213882, -29.706046) (-40.213882, -30.288929) (-40.806018, -30.288929) knots 0 0 0 1 1 1
  spline S21 degree 2 poles (-40.806018, -30.288929) (-41.398154, -30.288929) (-41.398154, -29.706046) knots 0 0 0 1 1 1
  line L155 (-41.398154, -29.706046) -> (-41.398154, -26.356778)
  line L156 (-41.398154, -26.356778) -> (-44.47911, -29.992861)
  spline S22 degree 2 poles (-44.47911, -29.992861) (-44.710413, -30.270425) (-44.950968, -30.270425) knots 0 0 0 1 1 1
  line L157 (-33.66338, -29.715298) -> (-33.66338, -22.248836)
  spline S23 degree 2 poles (-33.66338, -22.248836) (-33.66338, -21.656701) (-33.071244, -21.656701) knots 0 0 0 1 1 1
  line L158 (-33.071244, -21.656701) -> (-30.17533, -21.656701)
  spline S24 degree 2 poles (-30.17533, -21.656701) (-29.407404, -21.656701) (-28.34341, -22.729947) (-28.34341, -23.497873) knots 0 0 0 1 2 2 2
  line L159 (-28.34341, -23.497873) -> (-28.34341, -29.715298)
  spline S25 degree 2 poles (-28.34341, -29.715298) (-28.34341, -30.298181) (-28.935546, -30.298181) knots 0 0 0 1 1 1
  spline S26 degree 2 poles (-28.935546, -30.298181) (-29.527682, -30.298181) (-29.527682, -29.715298) knots 0 0 0 1 1 1
  line L160 (-29.527682, -29.715298) -> (-29.527682, -23.497873)
  spline S27 degree 2 poles (-29.527682, -23.497873) (-29.527682, -23.220309) (-29.916271, -22.83172) (-30.17533, -22.83172) knots 0 0 0 1 2 2 2
  line L161 (-30.17533, -22.83172) -> (-32.479108, -22.83172)
  line L162 (-32.479108, -22.83172) -> (-32.479108, -29.715298)
  spline S28 degree 2 poles (-32.479108, -29.715298) (-32.479108, -30.298181) (-33.071244, -30.298181) knots 0 0 0 1 1 1
  spline S29 degree 2 poles (-33.071244, -30.298181) (-33.66338, -30.298181) (-33.66338, -29.715298) knots 0 0 0 1 1 1
  line L163 (-26.872323, -29.706046) -> (-26.872323, -22.248836)
  spline S30 degree 2 poles (-26.872323, -22.248836) (-26.872323, -21.656701) (-26.280187, -21.656701) knots 0 0 0 1 1 1
  spline S31 degree 2 poles (-26.280187, -21.656701) (-25.688052, -21.656701) (-25.688052, -22.248836) knots 0 0 0 1 1 1
  line L164 (-25.688052, -22.248836) -> (-25.688052, -29.706046)
  spline S32 degree 2 poles (-25.688052, -29.706046) (-25.688052, -30.288929) (-26.280187, -30.288929) knots 0 0 0 1 1 1
  spline S33 degree 2 poles (-26.280187, -30.288929) (-26.872323, -30.288929) (-26.872323, -29.706046) knots 0 0 0 1 1 1
  line L165 (-19.26708, -28.466261) -> (-19.26708, -23.488621)
  spline S34 degree 2 poles (-19.26708, -23.488621) (-19.26708, -22.739199) (-18.193834, -21.656701) (-17.416656, -21.656701) knots 0 0 0 1 2 2 2
  line L166 (-17.416656, -21.656701) -> (-15.77903, -21.656701)
  spline S35 degree 2 poles (-15.77903, -21.656701) (-15.001852, -21.656701) (-13.928606, -22.729947) (-13.928606, -23.488621) knots 0 0 0 1 2 2 2
  line L167 (-13.928606, -23.488621) -> (-13.928606, -31.787773)
  spline S36 degree 2 poles (-13.928606, -31.787773) (-13.928606, -32.638968) (-14.502238, -33.138582) knots 0 0 0 1 1 1
  spline S37 degree 2 poles (-14.502238, -33.138582) (-15.011104, -33.601188) (-15.760526, -33.601188) knots 0 0 0 1 1 1
  spline S38 degree 2 poles (-15.760526, -33.601188) (-16.500696, -33.601188) (-17.018815, -33.138582) knots 0 0 0 1 1 1
  spline S39 degree 2 poles (-17.018815, -33.138582) (-17.592446, -32.629716) (-17.592446, -31.778521) knots 0 0 0 1 1 1
  spline S40 degree 2 poles (-17.592446, -31.778521) (-17.592446, -31.130872) (-17.166849, -30.622006) knots 0 0 0 1 1 1
  spline S41 degree 2 poles (-17.166849, -30.622006) (-16.815268, -30.33519) (-16.463687, -30.288929) knots 0 0 0 1 1 1
  line L168 (-16.463687, -30.288929) -> (-17.416656, -30.288929)
  spline S42 degree 2 poles (-17.416656, -30.288929) (-18.193834, -30.288929) (-19.26708, -29.215683) (-19.26708, -28.466261) knots 0 0 0 1 2 2 2
  line L169 (-12.476023, -28.466261) -> (-12.476023, -23.488621)
  spline S43 degree 2 poles (-12.476023, -23.488621) (-12.476023, -22.729947) (-11.402777, -21.656701) (-10.644104, -21.656701) knots 0 0 0 1 2 2 2
  line L170 (-10.644104, -21.656701) -> (-8.987974, -21.656701)
  spline S44 degree 2 poles (-8.987974, -21.656701) (-8.220048, -21.656701) (-7.156054, -22.729947) (-7.156054, -23.488621) knots 0 0 0 1 2 2 2
  line L171 (-7.156054, -23.488621) -> (-7.156054, -28.466261)
  spline S45 degree 2 poles (-7.156054, -28.466261) (-7.156054, -29.215683) (-8.2293, -30.288929) (-8.987974, -30.288929) knots 0 0 0 1 2 2 2
  line L172 (-8.987974, -30.288929) -> (-10.644104, -30.288929)
  spline S46 degree 2 poles (-10.644104, -30.288929) (-11.393525, -30.288929) (-12.476023, -29.206431) (-12.476023, -28.466261) knots 0 0 0 1 2 2 2
  line L173 (1.078333, -28.466261) -> (1.078333, -23.488621)
  spline S47 degree 2 poles (1.078333, -23.488621) (1.078333, -22.739199) (2.151579, -21.656701) (2.928757, -21.656701) knots 0 0 0 1 2 2 2
  line L174 (2.928757, -21.656701) -> (4.566383, -21.656701)
  spline S48 degree 2 poles (4.566383, -21.656701) (5.343561, -21.656701) (6.416807, -22.729947) (6.416807, -23.488621) knots 0 0 0 1 2 2 2
  line L175 (6.416807, -23.488621) -> (6.416807, -31.787773)
  spline S49 degree 2 poles (6.416807, -31.787773) (6.416807, -32.638968) (5.843175, -33.138582) knots 0 0 0 1 1 1
  spline S50 degree 2 poles (5.843175, -33.138582) (5.334309, -33.601188) (4.584887, -33.601188) knots 0 0 0 1 1 1
  spline S51 degree 2 poles (4.584887, -33.601188) (3.844717, -33.601188) (3.326599, -33.138582) knots 0 0 0 1 1 1
  spline S52 degree 2 poles (3.326599, -33.138582) (2.752967, -32.629716) (2.752967, -31.778521) knots 0 0 0 1 1 1
  spline S53 degree 2 poles (2.752967, -31.778521) (2.752967, -31.130872) (3.178565, -30.622006) knots 0 0 0 1 1 1
  spline S54 degree 2 poles (3.178565, -30.622006) (3.530145, -30.33519) (3.881726, -30.288929) knots 0 0 0 1 1 1
  line L176 (3.881726, -30.288929) -> (2.928757, -30.288929)
  spline S55 degree 2 poles (2.928757, -30.288929) (2.151579, -30.288929) (1.078333, -29.215683) (1.078333, -28.466261) knots 0 0 0 1 2 2 2
  line L177 (14.641942, -29.706046) -> (14.641942, -22.248836)
  spline S56 degree 2 poles (14.641942, -22.248836) (14.641942, -21.656701) (15.234078, -21.656701) knots 0 0 0 1 1 1
  spline S57 degree 2 poles (15.234078, -21.656701) (15.826214, -21.656701) (15.826214, -22.248836) knots 0 0 0 1 1 1
  line L178 (15.826214, -22.248836) -> (15.826214, -29.11391)
  line L179 (15.826214, -29.11391) -> (17.25104, -29.11391)
  line L180 (17.25104, -29.11391) -> (18.823901, -22.054542)
  spline S58 degree 2 poles (18.823901, -22.054542) (18.916422, -21.656701) (19.379028, -21.656701) knots 0 0 0 1 1 1
  spline S59 degree 2 poles (19.379028, -21.656701) (19.971164, -21.656701) (19.971164, -22.230332) knots 0 0 0 1 1 1
  spline S60 degree 2 poles (19.971164, -22.230332) (19.971164, -22.304349) (19.961912, -22.359862) knots 0 0 0 1 1 1
  line L181 (19.961912, -22.359862) -> (18.287278, -29.90034)
  spline S61 degree 2 poles (18.287278, -29.90034) (18.194757, -30.288929) (17.722898, -30.288929) knots 0 0 0 1 1 1
  line L182 (17.722898, -30.288929) -> (15.234078, -30.288929)
  spline S62 degree 2 poles (15.234078, -30.288929) (14.641942, -30.288929) (14.641942, -29.706046) knots 0 0 0 1 1 1
  line L183 (21.432999, -30.955082) -> (21.432999, -24.321311)
  spline S63 degree 2 poles (21.432999, -24.321311) (21.432999, -23.211057) (22.996607, -21.656701) (24.106862, -21.656701) knots 0 0 0 1 2 2 2
  line L184 (24.106862, -21.656701) -> (24.9303, -21.656701)
  spline S64 degree 2 poles (24.9303, -21.656701) (26.040555, -21.656701) (27.594911, -23.211057) (27.594911, -24.321311) knots 0 0 0 1 2 2 2
  line L185 (27.594911, -24.321311) -> (27.594911, -30.955082)
  spline S65 degree 2 poles (27.594911, -30.955082) (27.594911, -32.056084) (26.040555, -33.610441) (24.9303, -33.610441) knots 0 0 0 1 2 2 2
  line L186 (24.9303, -33.610441) -> (24.106862, -33.610441)
  spline S66 degree 2 poles (24.106862, -33.610441) (22.996607, -33.610441) (21.432999, -32.056084) (21.432999, -30.955082) knots 0 0 0 1 2 2 2
  line L187 (7.86939, -29.706046) -> (7.86939, -22.248836)
  spline S67 degree 2 poles (7.86939, -22.248836) (7.86939, -21.656701) (8.461526, -21.656701) knots 0 0 0 1 1 1
  line L188 (8.461526, -21.656701) -> (11.357439, -21.656701)
  spline S68 degree 2 poles (11.357439, -21.656701) (12.125365, -21.656701) (13.189359, -22.729947) (13.189359, -23.488621) knots 0 0 0 1 2 2 2
  line L189 (13.189359, -23.488621) -> (13.189359, -29.706046)
  spline S69 degree 2 poles (13.189359, -29.706046) (13.189359, -30.288929) (12.597224, -30.288929) knots 0 0 0 1 1 1
  spline S70 degree 2 poles (12.597224, -30.288929) (12.005088, -30.288929) (12.005088, -29.706046) knots 0 0 0 1 1 1
  line L190 (12.005088, -29.706046) -> (12.005088, -23.497873)
  spline S71 degree 2 poles (12.005088, -23.497873) (12.005088, -23.220309) (11.616499, -22.83172) (11.357439, -22.83172) knots 0 0 0 1 2 2 2
  line L191 (11.357439, -22.83172) -> (9.053661, -22.83172)
  line L192 (9.053661, -22.83172) -> (9.053661, -29.706046)
  spline S72 degree 2 poles (9.053661, -29.706046) (9.053661, -30.288929) (8.461526, -30.288929) knots 0 0 0 1 1 1
  spline S73 degree 2 poles (8.461526, -30.288929) (7.86939, -30.288929) (7.86939, -29.706046) knots 0 0 0 1 1 1
  spline S74 degree 2 poles (-5.111335, -30.270425) (-5.361143, -30.270425) (-5.721975, -29.909592) (-5.721975, -29.678289) knots 0 0 0 1 2 2 2
  spline S75 degree 2 poles (-5.721975, -29.678289) (-5.721975, -29.46549) (-5.564689, -29.2897) knots 0 0 0 1 1 1
  spline S76 degree 2 poles (-5.564689, -29.2897) (-4.269392, -27.864874) (-3.03886, -26.560325) knots 0 0 0 1 1 1
  line L193 (-3.03886, -26.560325) -> (-5.61095, -22.554156)
  spline S77 degree 2 poles (-5.61095, -22.554156) (-5.703471, -22.406122) (-5.703471, -22.248836) knots 0 0 0 1 1 1
  spline S78 degree 2 poles (-5.703471, -22.248836) (-5.703471, -21.999029) (-5.333386, -21.656701) (-5.102083, -21.656701) knots 0 0 0 1 2 2 2
  spline S79 degree 2 poles (-5.102083, -21.656701) (-4.796763, -21.656701) (-4.593217, -22.063794) knots 0 0 0 1 1 1
  line L194 (-4.593217, -22.063794) -> (-2.261682, -25.764642)
  spline S80 degree 2 poles (-2.261682, -25.764642) (-2.187665, -25.561096) (-1.558521, -24.867187) knots 0 0 0 1 1 1
  line L195 (-1.558521, -24.867187) -> (-1.558521, -22.248836)
  spline S81 degree 2 poles (-1.558521, -22.248836) (-1.558521, -21.656701) (-0.966385, -21.656701) knots 0 0 0 1 1 1
  spline S82 degree 2 poles (-0.966385, -21.656701) (-0.37425, -21.656701) (-0.37425, -22.248836) knots 0 0 0 1 1 1
  line L196 (-0.37425, -22.248836) -> (-0.37425, -29.706046)
  spline S83 degree 2 poles (-0.37425, -29.706046) (-0.37425, -30.288929) (-0.966385, -30.288929) knots 0 0 0 1 1 1
  spline S84 degree 2 poles (-0.966385, -30.288929) (-1.558521, -30.288929) (-1.558521, -29.706046) knots 0 0 0 1 1 1
  line L197 (-1.558521, -29.706046) -> (-1.558521, -26.356778)
  line L198 (-1.558521, -26.356778) -> (-4.639477, -29.992861)
  spline S85 degree 2 poles (-4.639477, -29.992861) (-4.87078, -30.270425) (-5.111335, -30.270425) knots 0 0 0 1 1 1
  line L199 (-25.216194, -24.737657) -> (-25.216194, -23.488621)
  spline S86 degree 2 poles (-25.216194, -23.488621) (-25.216194, -22.729947) (-24.142948, -21.656701) (-23.375022, -21.656701) knots 0 0 0 1 2 2 2
  line L200 (-23.375022, -21.656701) -> (-21.302547, -21.656701)
  spline S87 degree 2 poles (-21.302547, -21.656701) (-20.710411, -21.656701) (-20.710411, -22.248836) knots 0 0 0 1 1 1
  line L201 (-20.710411, -22.248836) -> (-20.710411, -29.706046)
  spline S88 degree 2 poles (-20.710411, -29.706046) (-20.710411, -30.288929) (-21.302547, -30.288929) knots 0 0 0 1 1 1
  spline S89 degree 2 poles (-21.302547, -30.288929) (-21.894682, -30.288929) (-21.894682, -29.706046) knots 0 0 0 1 1 1
  line L202 (-21.894682, -29.706046) -> (-21.894682, -26.560325)
  line L203 (-21.894682, -26.560325) -> (-23.384274, -26.560325)
  spline S90 degree 2 poles (-23.384274, -26.560325) (-24.142948, -26.560325) (-25.216194, -25.477826) (-25.216194, -24.737657) knots 0 0 0 1 2 2 2
  spline S91 degree 2 poles (-32.414343, -33.027557) (-32.414343, -32.435421) (-31.822208, -32.435421) knots 0 0 0 1 1 1
  line L204 (-31.822208, -32.435421) -> (-30.184582, -32.435421)
  spline S92 degree 2 poles (-30.184582, -32.435421) (-29.592447, -32.435421) (-29.592447, -33.027557) knots 0 0 0 1 1 1
  spline S93 degree 2 poles (-29.592447, -33.027557) (-29.592447, -33.610441) (-30.184582, -33.610441) knots 0 0 0 1 1 1
  line L205 (-30.184582, -33.610441) -> (-31.822208, -33.610441)
  spline S94 degree 2 poles (-31.822208, -33.610441) (-32.414343, -33.610441) (-32.414343, -33.027557) knots 0 0 0 1 1 1
  spline S95 degree 2 poles (-52.676489, -22.776207) (-53.083582, -22.618921) (-53.083582, -22.239584) knots 0 0 0 1 1 1
  spline S96 degree 2 poles (-53.083582, -22.239584) (-53.083582, -21.628944) (-52.500698, -21.628944) knots 0 0 0 1 1 1
  spline S97 degree 2 poles (-52.500698, -21.628944) (-52.065849, -21.628944) (-51.630999, -22.211828) knots 0 0 0 1 1 1
  spline S98 degree 2 poles (-51.630999, -22.211828) (-51.223906, -21.656701) (-50.391215, -21.656701) knots 0 0 0 1 1 1
  line L206 (-50.391215, -21.656701) -> (-48.735085, -21.656701)
  spline S99 degree 2 poles (-48.735085, -21.656701) (-47.967159, -21.656701) (-46.903165, -22.729947) (-46.903165, -23.488621) knots 0 0 0 1 2 2 2
  line L207 (-46.903165, -23.488621) -> (-46.903165, -28.466261)